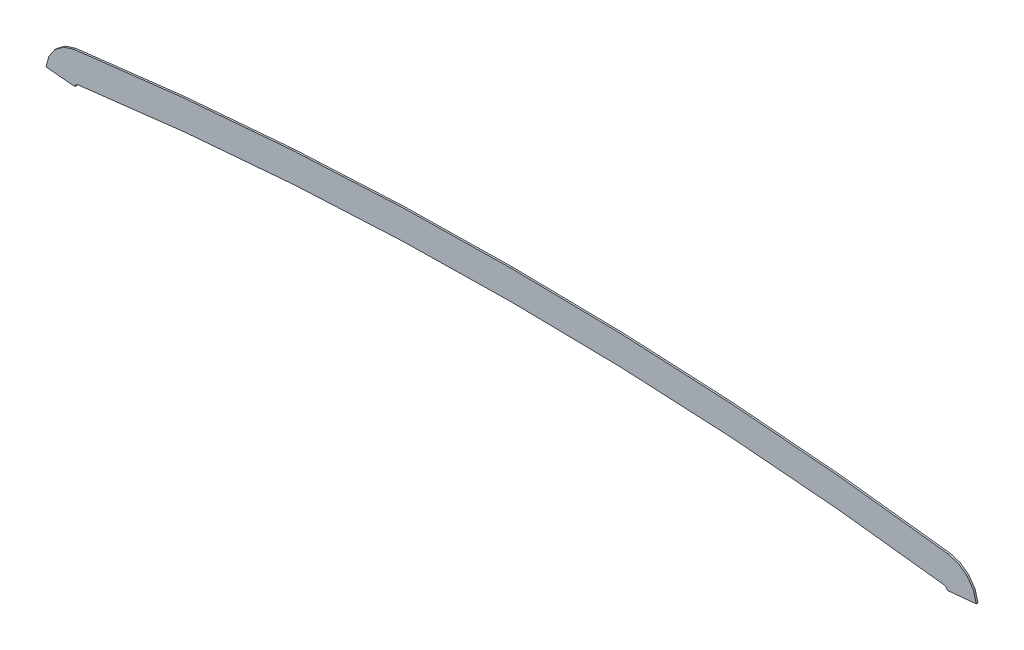
# Autodesk Inventor part: МОО 031 Усилитель спина
Saved by Autodesk Inventor 2024.2 (Build 282272000, 272)
## iProperties
Created: 2024-06-05
Part Number: МОО 031 Усилитель спина
Material: Generic
Document SubType Name: Sheet Metal
Designer: pokla
Density: 1 g/cm^3
Sheet Metal Rule: Default
Appearance: Default
Author: pokla
Autodesk Inventor part; units mm, degrees
ref_plane "YZ Plane" through (0, 0, 0) normal (1, 0, 0) x (0, 1, 0)
ref_plane "XZ Plane" through (0, 0, 0) normal (0, 1, 0) x (-1, 0, 0)
ref_plane "XY Plane" through (0, 0, 0) normal (0, 0, 1) x (1, 0, 0)
sketch "Sketch1" plane through (0, 0, 0) normal (0, 0, 1) x (1, 0, 0)
  line L0 (-750, 0) -> (750, 0) construction
  line L1 (750, 0) -> (750, -2700) construction
  line L2 (750, -2700) -> (-750, -2700) construction
  line L3 (-750, -2700) -> (-750, 0) construction
  line L4 (800, 50) -> (-800, 50) construction
  line L5 (-800, 50) -> (-800, -2750) construction
  line L6 (-800, -2750) -> (800, -2750) construction
  line L7 (800, -2750) -> (800, 50) construction
  line L8 (-850, 100) -> (850, 100) construction
  line L9 (850, 100) -> (850, -2800) construction
  line L10 (850, -2800) -> (-850, -2800) construction
  line L11 (-850, -2800) -> (-850, 100) construction
  arc A0 (750, 0) -> (745.2706, 0.6314) centre (0, -5600) ccw construction
  line L12 (-750, -2100) -> (750, -2100) construction
  line L13 (114.1118, -2698.3696) -> (750, -2100) construction
  arc A1 (750, -2100) -> (768.2917, -213.4901) centre (-10250, -1050) ccw construction
  line L14 (750, 0) -> (749.6018, -2.9735) construction
  arc A2 (750, -3.0268) -> (0, 47) centre (-0.2, -5603) ccw construction
  line L15 (750, 0) -> (747.0136, -0.2851) construction
  arc A3 (767.1641, -238.6409) -> (747.4657, -5.0326) centre (-10252.9895, -1050.2527) ccw construction
  arc A4 (750.4522, -4.7486) -> (745.2706, 0.6314) centre (744.4791, -5.3162) ccw
  arc A5 (747.4657, -5.0326) -> (744.8748, -2.3426) centre (744.4792, -5.3164) ccw construction
  line L16 (750, -2100) -> (752.9864, -2100.2851) construction
  arc A6 (752.9864, -2100.2851) -> (803.0109, -1050.0292) centre (-10246.9891, -1050.0292) ccw construction
  line L17 (750, -2100) -> (752.0559, -2102.1848) construction
  line L18 (752.0559, -2102.1848) -> (752.0559, -2102.1848) construction
  arc A7 (749.1768, -2100.7746) -> (750.1074, -2098.8746) centre (747.1209, -2098.5898) ccw construction
  line L19 (0, -2697) -> (110, -2697) construction
  line L20 (112.0559, -2696.1848) -> (690.4112, -2151.9536) construction
  arc A8 (110, -2700) -> (114.1118, -2698.3696) centre (110, -2694) ccw construction
  arc A9 (110, -2697) -> (112.0559, -2696.1848) centre (110, -2694) ccw construction
  line L21 (690.4112, -2151.9536) -> (692.4671, -2154.1384) construction
  line L22 (752.0559, -2102.1848) -> (676.3163, -2173.4556) construction
  line L23 (676.3163, -2173.4556) -> (674.2605, -2171.2708) construction
  arc A10 (747.4657, -5.0326) -> (747.0136, -0.2851) centre (-10252.9895, -1050.2527) ccw construction
  arc A11 (745.2706, 0.6314) -> (0, 50) centre (0, -5600) ccw
  arc A12 (750.4522, -4.7486) -> (750, 0) centre (-10250, -1050) ccw construction
  line L24 (770.156, -238.4205) -> (767.1641, -238.6409) construction
  line L25 (768.2917, -213.4901) -> (771.2831, -213.263) construction
  arc A13 (768.2917, -213.4901) -> (750.4522, -4.7486) centre (-10250, -1050) ccw construction
  line L26 (0, 100) -> (0, 50) construction
  line L27 (0, -2700) -> (0, -2697) construction
  line L28 (0, 47) -> (0, 0) construction
  line L29 (0, 50) -> (0, 47) construction
  arc A14 (752.0559, -2102.1848) -> (752.9864, -2100.2851) centre (749.9998, -2099.9999) ccw construction
  arc A15 (803.0109, -1050.0292) -> (771.2831, -213.263) centre (-10246.9891, -1050.0292) ccw construction
  line L30 (0, 50) -> (0, 100)
  line L31 (745.2706, 0.6314) -> (751.8659, 50.1945) construction
  line L32 (750.4522, -4.7486) -> (800.228, -0.019)
  arc A16 (751.8659, 50.1945) -> (0, 100) centre (3.3122, -5549.999) ccw
  arc A17 (800.228, -0.019) -> (751.8659, 50.1945) centre (744.4411, -5.3528) ccw
  line L33 (767.1641, -238.6409) -> (817.0291, -234.9684) construction
  arc A18 (817.0291, -234.9684) -> (800.228, -0.019) centre (-10212.6009, -905.6121) ccw construction
  line L34 (800, -1050) -> (850, -1050) construction
  line L35 (750.1074, -2098.8746) -> (799.8816, -2103.6206) construction
  line L36 (749.1768, -2100.7746) -> (783.4416, -2137.1879) construction
  line L37 (114.1118, -2698.3696) -> (148.3766, -2734.7828) construction
  line L38 (110, -2700) -> (110, -2750) construction
  line L39 (110, -2700) -> (0, -2700) construction
  line L40 (0, -2700) -> (0, -2750) construction
  arc A19 (850, -1050) -> (817.0291, -234.9684) centre (-10199.9318, -1088.8264) ccw construction
  arc A20 (799.8816, -2103.6206) -> (850, -1050) centre (-10199.9997, -1052.3784) ccw construction
  arc A21 (783.4416, -2137.1879) -> (799.8816, -2103.6206) centre (747.0918, -2098.5756) ccw construction
  line L41 (783.4416, -2137.1879) -> (148.3766, -2734.7828) construction
  line L42 (110, -2750) -> (0, -2750) construction
  arc A22 (110, -2750) -> (148.3766, -2734.7828) centre (110, -2694) ccw construction
  point P0 (0, -2750)
  dimension "d0" = 1500
  dimension "d1" = 2700
  dimension "d2" = 2100
  dimension "d3" = 6
  dimension "d4" = 3
  dimension "d5" = 3
  dimension "d6" = 6
  dimension "d7" = 3
  dimension "d8" = 239.271
  dimension "d9" = 50
  dimension "d10" = 50
  dimension "d11" = 3
  dimension "d12" = 25
  dimension "d13" = 110
  dimension "d14" = 25
  dimension "d15" = 104
  dimension "d28" = 50
  constraints: 87 end point, 52 point on circle, 23 centre point, 18 equal length, 18 tangent, 16 line through centre, 13 perpendicular, 8 parallel, 8 point on line, 7 equal radius, 5 midpoint, 4 vertical, 2 coincident, 2 horizontal, 1 collinear, 6 other
  measures "d0" distance of L0.start L15.start
  measures "d1" distance of L15.start L1.end
  measures "d2" distance between parallel lines of L12 L0
  measures "d3" radius of A4
  measures "d4" radius of A5
  measures "d5" radius of A7
  measures "d6" radius of A8
  measures "d7" radius of A9
  measures "d8" distance of L15.start L24.start
  measures "d9" distance between parallel lines of L4 L8
  measures "d10" distance between parallel lines of L0 L4
  measures "d11" distance of L29.start L28.start
  measures "d12" distance of L24.start L25.start
  measures "d13" distance from line of L27 A8.centre
  measures "d14" distance of L23.end L21.end
  measures "d15" distance of L17.start L23.end
  measures "d28" distance of L29.start L30.end
extrude "Extrusion1" add sketch "Sketch1" along normal mid plane 3
mirror "Mirror1" about plane through (0, 0, 0) normal (1, 0, 0) of "Extrusion1"
equation "\"d0\" = Бак_ширина_общая"
equation "\"d1\" = Бак_высота_общая"
equation "\"d2\" = Бак_высота_до_конуса"
equation "\"d3\" = Thickness + BendRadius"
equation "\"d4\" = Thickness"
equation "\"d5\" = Thickness"
equation "\"d6\" = Thickness + BendRadius"
equation "\"d7\" = Thickness"
equation "\"d8\" = Бак_спина_длина_фланцев"
equation "\"d11\" = d21"
equation "\"d12\" = Бак_нахлест_фланца"
equation "\"d13\" = 0.5 * Бак_брюхо_ширина_полки"
equation "\"d14\" = Бак_нахлест_фланца"
equation "\"d15\" = Бак_борт_длина_фланца"
equation "\"d19\" = d21 + d25"
equation "\"d20\" = d21"
equation "\"d25\" = d21"
equation "\"BendRadius\" = Thickness"
equation "\"BendReliefWidth\" = Thickness"
equation "\"BendReliefDepth\" = 0.5 * Thickness"
equation "\"CornerReliefSize\" = 4 * Thickness"
equation "\"MinimumRemnant\" = 2 * Thickness"
equation "\"TransitionRadius\" = BendRadius"
equation "\"JacobiRadiusSize\" = BendRadius"
equation "\"GapSize\" = Thickness"
equation "\"Бак_ширина_общая\" = 1500"
equation "\"Бак_высота_общая\" = 2700"
equation "\"Бак_высота_до_конуса\" = 2100"
equation "\"Thickness\" = 3"
equation "\"Бак_спина_длина_фланцев\" = 239.271"
equation "\"d21\" = 3"
equation "\"Бак_нахлест_фланца\" = 25"
equation "\"Бак_брюхо_ширина_полки\" = 220"
equation "\"Бак_борт_длина_фланца\" = 104"
body "Solid1"
